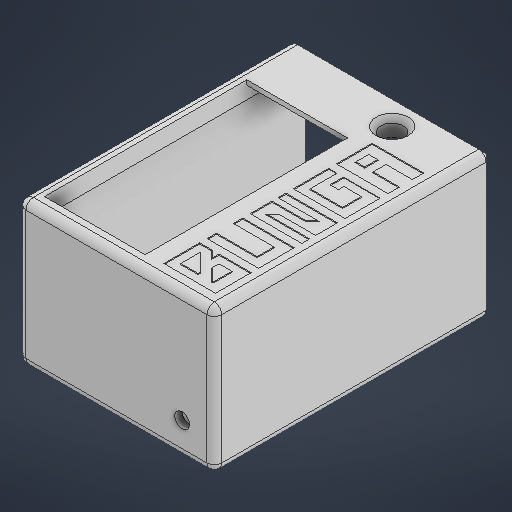
# Autodesk Inventor part: PowerSupplyRegulator-OnePiece
Saved by Autodesk Inventor 2026.2 (Build 302298010, 298A)
## iProperties
Created: 2026-07-26
Part Number: PowerSupplyRegulator-OnePiece
Material: Generic
Document SubType Name: Modeling
Designer: incep
Density: 1 g/cm^3
Appearance: Default
Author: incep
## iProperties of the stored document PowerSupplyRegulator-OnePiece_3DPrint.ipt
Created: 2026-07-26
Part Number: PowerSupplyRegulator-OnePiece_3DPrint
Material: Generic
Document SubType Name: Modeling
Designer: incep
Density: 1 g/cm^3
Appearance: Default
Author: incep
Autodesk Inventor part; units mm, degrees
ref_plane "YZ Plane" through (0, 0, 0) normal (1, 0, 0) x (0, 1, 0)
ref_plane "XZ Plane" through (0, 0, 0) normal (0, 1, 0) x (-1, 0, 0)
ref_plane "XY Plane" through (0, 0, 0) normal (0, 0, 1) x (1, 0, 0)
sketch "Sketch1" plane through (0, 0, 0) normal (0, 0, 1) x (1, 0, 0)
  line L0 (-36.5, 21.9) -> (36.5, 21.9)
  line L1 (36.5, 21.9) -> (36.5, -21.9)
  line L2 (36.5, -21.9) -> (-36.5, -21.9)
  line L3 (-36.5, -21.9) -> (-36.5, 21.9)
  line L4 (-39.5, 28.9) -> (39.5, 28.9)
  line L5 (39.5, 28.9) -> (39.5, -28.9)
  line L6 (39.5, -28.9) -> (-39.5, -28.9)
  line L7 (-39.5, -28.9) -> (-39.5, 28.9)
  point P0 (0, 0)
  point P1 (36.5, 0)
  point P2 (0, 21.9)
  point P3 (0, 28.9)
  point P4 (39.5, 0)
  dimension "d0" = 73
  dimension "d1" = 43.8
  dimension "d2" = 3
  dimension "d3" = 7
  constraints: 16 end point, 4 midpoint, 4 parallel, 2 horizontal, 2 horizontal alignment, 2 perpendicular, 2 vertical alignment
  measures "d0" distance of L0.start L0.end
  measures "d1" distance of L2.end L0.start
  measures "d2" distance between parallel lines of L7 L3
  measures "d3" distance between parallel lines of L4 L0
extrude "Extrusion1" add sketch "Sketch1" along normal blind 109.6
sketch "Sketch3" plane through (0, 0, 109.6) normal (0, 0, 1) x (1, 0, 0)
  point P0 (0, 0)
sketch "Sketch2" plane through (0, 0, 109.6) normal (0, 0, 1) x (1, 0, 0)
  line L0 (39.5, -28.9) -> (39.5, 28.9) projected
  line L1 (39.5, 28.9) -> (-39.5, 28.9) projected
  line L2 (-39.5, 28.9) -> (-39.5, -28.9) projected
  line L3 (-39.5, -28.9) -> (39.5, -28.9) projected
  point P0 (0, 0)
sketch "Sketch4" plane through (0, 0, 109.6) normal (0, 0, 1) x (1, 0, 0)
  line L0 (-36.5, 27) -> (36.5, 27)
  line L1 (36.5, 27) -> (36.5, -27)
  line L2 (36.5, -27) -> (-36.5, -27)
  line L3 (-36.5, -27) -> (-36.5, 27)
  line L4 (-36.5, -21.9) -> (-36.5, 21.9) projected
  line L5 (39.5, 28.9) -> (-39.5, 28.9) projected
  point P0 (0, 0)
  point P1 (36.5, 0)
  point P2 (0, 27)
  dimension "d6" = 54
  dimension "d43" = 1.9
  constraints: 8 end point, 2 midpoint, 2 parallel, 1 collinear, 1 horizontal, 1 horizontal alignment, 1 perpendicular, 1 vertical alignment
  measures "d6" distance between parallel lines of L2 L0
  measures "d43" distance between parallel lines of L5 L0
extrude "Extrusion2" cut sketch "Sketch4" against normal blind 86.6
sketch "Sketch6" plane through (-39.5, 28.9, 0) normal (0, 1, 0) x (1, 0, 0)
  line L0 (3, -109.6) -> (76, -109.6) projected
  line L1 (3, -109.6) -> (3, -23) projected
  line L2 (3, -23) -> (76, -23) projected
  line L3 (76, -109.6) -> (76, -23) projected
  line L4 (45.6, -25.5) -> (5, -25.5)
  line L5 (5, -25.5) -> (5, -107.1)
  line L6 (5, -107.1) -> (45.6, -107.1)
  line L7 (45.6, -107.1) -> (45.6, -25.5)
  point P0 (39.5, 0)
  point P1 (45.6, -66.3)
  point P2 (76, -66.3)
  point P3 (25.3, -25.5)
  point P4 (39.5, -23)
  dimension "d9" = 81.6
  dimension "d10" = 40.6
  dimension "d11" = 2
  dimension "d20" = 2.5
  constraints: 8 end point, 4 midpoint, 2 parallel, 1 horizontal, 1 perpendicular
  measures "d9" distance of L6.end L4.start
  measures "d10" distance between parallel lines of L5 L7
  measures "d11" distance between parallel lines of L1 L5
  measures "d20" distance between parallel lines of L0 L6
extrude "Extrusion3" cut sketch "Sketch6" against normal up to surface (1.9 mm away) contours L7 L6 L5 L4
sketch "Sketch7" plane through (-36.5, -21.9, 0) normal (0, 1, 0) x (1, 0, 0)
  circle A0 centre (62.3, -14.3) radius 5.25
  circle A1 centre (10.7, -14.3) radius 5.25
  line L0 (62.3, -14.3) -> (10.7, -14.3) construction
  line L1 (73, 0) -> (0, 0) construction
  point P0 (36.5, 0)
  point P1 (36.5, 0)
  point P2 (36.5, -14.3)
  dimension "d14" = 51.6
  dimension "d15" = 10.5
  dimension "d16" = 14.3
  constraints: 2 centre point, 2 end point, 2 midpoint, 1 equal radius, 1 horizontal, 1 vertical alignment
  measures "d14" distance of L0.start L0.end
  measures "d15" diameter of A0
  measures "d16" distance between parallel lines of L0 L1
extrude "Extrusion4" cut sketch "Sketch7" against normal blind 0.9
fillet "Fillet1" [suppressed]
chamfer "Chamfer1" distance 3 angle 45 2 edges at (0, 21.9, 23) (0, -21.9, 23)
chamfer "Chamfer2" distance 2 angle 45 1 edges at (0, -21.9, 0)
sketch "Sketch8" plane through (-39.5, -25.95, 0) normal (-1, 0, 0) x (0, 0, 1)
  line L0 (2, 4.05) -> (20, 4.05) projected
  line L1 (2, 4.05) -> (20, 4.05) projected
  line L2 (9.05, 4.05) -> (19.55, 4.05) projected
  line L3 (9.05, 4.05) -> (19.55, 4.05) projected
  circle A0 centre (8.5, 1) radius 2.1
  line L4 (0, -2.95) -> (109.6, -2.95) projected
  line L5 (0, -2.95) -> (109.6, -2.95) projected
  point P0 (0, 25.95)
  point P1 (8.5, 4)
  point P2 (8.5, 4)
  dimension "d27" = 4.2
  dimension "d28" = 3
  constraints: 1 centre point, 1 vertical alignment, 4 other
  measures "d27" diameter of A0
  measures "d28" distance of A0.centre point (8.5, 4)
extrude "Extrusion5" [suppressed]
sketch "Sketch9" plane through (-33.5, -24.95, 8.5) normal (-1, 0, 0) x (0, 0, 1)
  circle A0 centre (0, 0) radius 2.1 projected
  circle A1 centre (0, 0) radius 1.7
  point P0 (-8.5, 24.95)
  dimension "d31" = 3.4
  constraints: 1 centre point, 1 coincident
  measures "d31" diameter of A1
extrude "Extrusion6" [suppressed]
sketch "Sketch10" plane through (39.5, -25.95, 0) normal (1, 0, 0) x (0, 0, -1)
  point P0 (0, 25.95)
sketch "Sketch11" plane through (39.5, -25.95, 0) normal (1, 0, 0) x (0, 0, -1)
  circle A0 centre (-8.5, 1) radius 1.7 projected
  circle A1 centre (-8.5, 1) radius 3
  point P0 (0, 25.95)
  dimension "d34" = 6
  constraints: 1 centre point, 1 coincident
  measures "d34" diameter of A1
extrude "Extrusion7" add sketch "Sketch2" along normal blind 3
fillet "Fillet2" [suppressed]
sketch "Sketch12" plane through (0, 0, 112.6) normal (0, 0, 1) x (1, 0, 0)
  circle A0 centre (26.5, -15.95) radius 3
  line L0 (36.5, 25.95) -> (36.5, -25.95) projected
  line L1 (36.5, -25.95) -> (-36.5, -25.95) projected
  point P0 (0, 0)
  dimension "d38" = 6
  dimension "d39" = 10
  dimension "d40" = 10
  constraints: 1 centre point
  measures "d38" diameter of A0
  measures "d39" distance from line of L0 A0.centre
  measures "d40" distance from line of L1 A0.centre
extrude "Extrusion8" cut sketch "Sketch12" against normal up to surface (3 mm away)
fillet "Fillet3" radius 3 8 edges at (-39.5, -28.9, 56.3) (-39.5, 28.9, 56.3) (39.5, -28.9, 56.3) (39.5, 28.9, 56.3) (0, 28.9, 112.6) (39.5, 0, 112.6) (0, -28.9, 112.6) (-39.5, 0, 112.6)
fillet "Fillet4" radius 6 4 edges at (36.5, -21.9, 11) (36.5, 21.9, 10) (-36.5, -21.9, 11) (-36.5, 21.9, 10)
sketch "Sketch13" plane through (-36.5, 28.9, 0) normal (0, 1, 0) x (1, 0, 0)
  line L0 (0, -23) -> (73, -23) projected
  line L1 (0, -14) -> (0, 0) projected
  line L2 (0, -23) -> (0, -14) projected
  line L3 (0, -109.6) -> (0, -23) projected
  line L4 (0, -109.6) -> (0, -23) projected
  line L5 (0, -14) -> (0, -23) projected
  line L6 (0, -8) -> (0, -14) projected
  line L7 (0, 0) -> (0, -8) projected
  line L8 (73, 0) -> (73, -14) projected
  line L9 (73, -8) -> (73, 0) projected
  line L10 (73, -14) -> (73, -8) projected
  line L11 (73, -23) -> (73, -14) projected
  line L12 (73, -109.6) -> (73, -23) projected
  line L13 (73, -109.6) -> (73, -23) projected
  line L14 (73, -14) -> (73, -23) projected
  circle A0 centre (47.6, -12.5) radius 4.5
  point P0 (36.5, 0)
  dimension "d46" = 9
  dimension "d47" = 25.4
  dimension "d48" = 10.5
  constraints: 1 centre point
  measures "d46" diameter of A0
  measures "d47" distance from line of A0.centre L11
  measures "d48" distance from line of L0 A0.centre
extrude "Extrusion9" cut sketch "Sketch13" against normal up to surface (7 mm away)
chamfer "Chamfer3" distance 2 angle 45 1 edges at (6.6, 28.9, 12.5)
chamfer "Chamfer4" distance 3 angle 45 8 edges at (0, 28.9, 0) (-38.6213, 28.0213, 0) (-39.5, 0, 0) (-38.6213, -28.0213, 0) (0, -28.9, 0) (38.6213, -28.0213, 0) (39.5, 0, 0) (38.6213, 28.0213, 0)
sketch "Sketch14" plane through (-36.5, 28.9, 109.6) normal (0, 1, 0) x (1, 0, 0)
  line L0 (70.0467, 55.6168) -> (49.6467, 55.6168) construction
  line L1 (49.6467, 52.2168) -> (70.0467, 52.2168) construction
  line L2 (49.6467, 55.6168) -> (49.6467, 69.6168) construction
  line L3 (49.6467, 55.6168) -> (70.0467, 55.6168)
  line L4 (49.6467, 69.6168) -> (49.6467, 55.6168)
  line L5 (70.0467, 69.6168) -> (70.0467, 55.6168) construction
  line L6 (49.6467, 69.6168) -> (70.0467, 69.6168) construction
  line L7 (70.0467, 55.6168) -> (49.6467, 55.6168) construction
  line L8 (55.6467, 64.4168) -> (58.6467, 64.4168)
  line L9 (58.6467, 64.4168) -> (58.6467, 66.6168)
  line L10 (66.0467, 66.6168) -> (66.0467, 58.6168)
  line L11 (58.6467, 66.6168) -> (66.0467, 66.6168)
  line L12 (52.6467, 58.6168) -> (52.6467, 69.6168)
  line L13 (55.6467, 69.6168) -> (55.6467, 64.4168)
  line L14 (70.0467, 55.6168) -> (70.0467, 69.6168)
  line L15 (70.0467, 69.6168) -> (55.6467, 69.6168)
  line L16 (66.0467, 58.6168) -> (52.6467, 58.6168)
  line L17 (49.6467, 69.6168) -> (70.0467, 69.6168) construction
  line L18 (70.0467, 73.0168) -> (49.6467, 73.0168) construction
  line L19 (49.6467, 87.0168) -> (70.0467, 87.0168) construction
  line L20 (49.6467, 73.0168) -> (49.6467, 87.0168) construction
  line L21 (70.0467, 87.0168) -> (70.0467, 73.0168) construction
  line L22 (52.6467, 69.6168) -> (49.6467, 69.6168)
  line L23 (49.6467, 73.0168) -> (70.0467, 73.0168)
  line L24 (70.0467, 73.0168) -> (70.0467, 77.2168)
  line L25 (70.0467, 77.2168) -> (59.4467, 77.2168)
  line L26 (52.4467, 77.2168) -> (56.4467, 77.2168)
  line L27 (59.4467, 77.2168) -> (59.4467, 82.8168)
  line L28 (59.4467, 82.8168) -> (70.0467, 82.8168)
  line L29 (70.0467, 82.8168) -> (70.0467, 87.0168)
  line L30 (70.0467, 87.0168) -> (49.6467, 87.0168)
  line L31 (49.6467, 87.0168) -> (49.6467, 73.0168)
  line L32 (56.4467, 82.8168) -> (52.4467, 82.8168)
  line L33 (52.4467, 82.8168) -> (52.4467, 77.2168)
  line L34 (56.4467, 77.2168) -> (56.4467, 82.8168)
  line L35 (70.0467, 38.2168) -> (49.6467, 38.2168) construction
  line L36 (49.6467, 34.8168) -> (70.0467, 34.8168) construction
  line L37 (49.6467, 34.8168) -> (70.0467, 34.8168) construction
  line L38 (70.0467, 34.8168) -> (70.0467, 20.8168) construction
  line L39 (70.0467, 20.8168) -> (49.6467, 20.8168) construction
  line L40 (49.6467, 20.8168) -> (49.6467, 34.8168) construction
  line L41 (49.6467, 20.8168) -> (49.6467, 34.8168) construction
  line L42 (70.0467, 52.2168) -> (70.0467, 38.2168) construction
  line L43 (49.6467, 38.2168) -> (49.6467, 52.2168) construction
  line L44 (49.6467, 52.2168) -> (70.0467, 52.2168) construction
  line L45 (70.0467, 38.2168) -> (49.6467, 38.2168) construction
  line L46 (70.0467, 52.2168) -> (70.0467, 38.2168) construction
  line L47 (49.6467, 38.2168) -> (49.6467, 52.2168) construction
  line L48 (49.6467, 55.6168) -> (49.6467, 69.6168) construction
  line L49 (70.0467, 69.6168) -> (70.0467, 55.6168) construction
  line L50 (49.6467, 38.2168) -> (49.6467, 52.2168) construction
  line L51 (70.0467, 41.0168) -> (70.0467, 38.2168)
  line L52 (55.4467, 43.8168) -> (52.6467, 41.0168)
  line L53 (49.6467, 46.6168) -> (63.2467, 46.6168)
  line L54 (66.0467, 49.4168) -> (49.6467, 49.4168)
  line L55 (49.6467, 52.2168) -> (70.0467, 52.2168) construction
  line L56 (49.6467, 52.2168) -> (70.0467, 52.2168)
  line L57 (70.0467, 38.2168) -> (49.6467, 38.2168)
  line L58 (70.0467, 38.2168) -> (49.6467, 38.2168) construction
  line L59 (52.6467, 41.0168) -> (70.0467, 41.0168)
  line L60 (70.0467, 43.8168) -> (55.4467, 43.8168)
  line L61 (63.2467, 46.6168) -> (66.0467, 49.4168)
  line L62 (70.0467, 52.2168) -> (70.0467, 38.2168) construction
  line L63 (70.0467, 52.2168) -> (70.0467, 43.8168)
  line L64 (70.0467, 34.8168) -> (70.0467, 20.8168) construction
  line L65 (59.8467, 15.3688) -> (59.8467, 15.3688)
  line L66 (49.6467, 17.4168) -> (54.4376, 17.4168)
  line L67 (53.171, 14.4168) -> (52.6467, 14.4168)
  line L68 (54.4376, 17.4168) -> (57.4376, 14.4168)
  line L69 (57.4376, 14.4168) -> (57.4376, 17.4168)
  line L70 (59.8467, 15.3688) -> (59.8467, 17.4168) construction
  line L71 (59.8467, 15.3688) -> (59.8467, 17.4168) construction
  line L72 (57.4376, 14.4168) -> (60.4376, 11.4168) construction
  line L73 (60.4376, 11.4168) -> (60.4376, 14.4168)
  line L74 (60.4376, 14.4168) -> (66.0467, 14.4168)
  line L75 (70.0467, 17.4168) -> (57.4376, 17.4168)
  line L76 (49.6467, 34.8168) -> (70.0467, 34.8168)
  line L77 (66.0467, 31.4168) -> (49.6467, 31.4168)
  line L78 (66.0467, 24.2168) -> (66.0467, 31.4168)
  line L79 (70.0467, 34.8168) -> (70.0467, 20.8168)
  line L80 (49.6467, 24.2168) -> (66.0467, 24.2168)
  line L81 (49.6467, 20.8168) -> (49.6467, 24.2168)
  line L82 (70.0467, 20.8168) -> (49.6467, 20.8168)
  line L83 (49.6467, 17.4168) -> (49.6467, 3.4168)
  line L84 (70.0467, 3.4168) -> (70.0467, 17.4168)
  line L85 (49.6467, 17.4168) -> (70.0467, 17.4168) construction
  line L86 (49.6467, 3.4168) -> (49.6467, 17.4168) construction
  line L87 (70.0467, 3.4168) -> (49.6467, 3.4168) construction
  line L88 (70.0467, 17.4168) -> (70.0467, 3.4168) construction
  line L89 (70.0467, 20.8168) -> (49.6467, 20.8168) construction
  line L90 (52.6467, 6.4168) -> (60.0715, 6.4168)
  line L91 (56.3591, 6.4168) -> (56.3591, 11.945) construction
  line L92 (60.0715, 6.4168) -> (60.0715, 7.5163)
  line L93 (66.0467, 14.4168) -> (66.0467, 6.4168)
  line L94 (66.0467, 6.4168) -> (65.4376, 6.4168)
  line L95 (65.4376, 6.4168) -> (60.4376, 11.4168)
  line L96 (60.0715, 7.5163) -> (53.171, 14.4168)
  line L97 (52.6467, 14.4168) -> (52.6467, 6.4168)
  line L98 (65.4376, 6.4168) -> (65.4376, 0.7147) construction
  line L99 (49.6467, 3.4168) -> (70.0467, 3.4168)
  line L100 (49.6467, 52.2168) -> (49.6467, 49.4168)
  line L101 (49.6467, 46.6168) -> (49.6467, 38.2168)
  line L102 (49.6467, 34.8168) -> (49.6467, 31.4168)
  point P0 (36.5, 109.6)
  point P1 (48.2467, 45.2168)
  point P2 (49.6467, 62.6168)
  point P3 (49.6467, 62.6168)
  point P4 (59.8467, 52.2168)
  point P5 (59.8467, 62.6168)
  point P6 (59.8467, 69.6168)
  point P7 (59.8467, 69.6168)
  point P8 (49.6467, 80.0168)
  point P9 (59.8467, 80.0168)
  point P10 (59.8467, 87.0168)
  point P11 (49.6467, 45.2168)
  point P12 (59.8467, 45.2168)
  point P13 (59.8467, 34.8168)
  point P14 (59.8467, 34.8168)
  point P15 (49.6467, 27.8168)
  point P16 (49.6467, 27.8168)
  point P17 (49.6467, 45.2168)
  point P18 (59.8467, 62.6168)
  point P19 (59.8467, 53.2168)
  point P20 (59.8467, 52.2168)
  point P21 (59.8467, 45.2168)
  point P22 (49.6467, 45.2168)
  point P23 (59.8467, 45.2168)
  point P24 (59.8467, 52.2168)
  point P25 (59.8467, 45.2168)
  point P26 (55.6986, 19.5168)
  point P27 (59.8467, 17.4168)
  point P28 (49.6467, 10.4168)
  point P29 (59.8467, 10.4168)
  point P30 (59.8467, 27.8168)
  point P31 (59.8467, 27.8168)
  point P32 (61.4467, 45.2168)
  point P33 (61.4467, 45.2168)
  constraints: 206 end point, 27 perpendicular, 17 collinear, 17 point on line, 6 midpoint, 4 parallel, 2 coincident
extrude "Extrusion10" cut sketch "Sketch14" against normal blind 0.2
chamfer "Chamfer5" distance 0.2 angle 45 58 edges at (13.1467, 28.9, 99.1832) (15.5421, 28.9, 92.1832) (23.3467, 28.9, 106.1832) (33.5467, 28.9, 99.1832) (27.2421, 28.9, 92.1832) (20.9376, 28.9, 93.6832) (19.4376, 28.9, 93.6832) (20.1212, 28.9, 98.6334) (23.5715, 28.9, 102.6334) (19.8591, 28.9, 103.1832) (16.1467, 28.9, 99.1832) (26.4376, 28.9, 100.6832) (23.9376, 28.9, 96.6832) (26.7421, 28.9, 95.1832) (29.5467, 28.9, 99.1832) (29.2421, 28.9, 103.1832) (23.3467, 28.9, 88.7832) (13.1467, 28.9, 87.0832) (21.3467, 28.9, 85.3832) (21.3467, 28.9, 78.1832) (13.1467, 28.9, 76.4832) (23.3467, 28.9, 74.7832) (33.5467, 28.9, 81.7832) (29.5467, 28.9, 81.7832) (13.1467, 28.9, 67.1832) (23.3467, 28.9, 71.3832) (24.8467, 28.9, 68.5832) (17.5467, 28.9, 67.1832) (26.2467, 28.9, 65.7832) (33.5467, 28.9, 69.9832) (33.5467, 28.9, 61.5832) (19.9467, 28.9, 62.9832) (28.1467, 28.9, 61.5832) (21.3467, 28.9, 60.1832) (13.1467, 28.9, 58.7832) (23.3467, 28.9, 57.3832) (13.1467, 28.9, 46.9832) (23.3467, 28.9, 53.9832) (22.8467, 28.9, 50.9832) (16.1467, 28.9, 45.4832) (19.1467, 28.9, 42.5832) (20.6467, 28.9, 45.1832) (22.1467, 28.9, 44.0832) (25.8467, 28.9, 42.9832) (29.5467, 28.9, 46.9832) (33.5467, 28.9, 46.9832) (23.3467, 28.9, 36.5832) (13.1467, 28.9, 29.5832) (23.3467, 28.9, 22.5832) (19.9467, 28.9, 29.5832) (17.9467, 28.9, 32.3832) (15.9467, 28.9, 29.5832) (17.9467, 28.9, 26.7832) (22.9467, 28.9, 29.5832) (28.2467, 28.9, 32.3832) (28.2467, 28.9, 26.7832) (33.5467, 28.9, 24.6832) (33.5467, 28.9, 34.4832)
sketch "Sketch15" plane through (-36.5, 27, 23) normal (0, -1, 0) x (1, 0, 0)
  line L0 (42.6, -3) -> (73, -3)
  line L1 (73, -3) -> (73, 86.6)
  line L2 (73, 86.6) -> (42.6, 86.6)
  line L3 (42.6, 86.6) -> (42.6, -3)
  line L4 (42.6, 84.1) -> (42.6, 2.5) projected
  line L5 (0, 86.6) -> (73, 86.6) projected
  line L6 (6, -3) -> (67, -3) projected
  line L7 (73, 86.6) -> (73, 0) projected
  line L8 (0, 86.6) -> (2, 86.6)
  line L9 (2, 86.6) -> (2, -3)
  line L10 (2, -3) -> (0, -3)
  line L11 (0, -3) -> (0, 86.6)
  line L12 (0, 86.6) -> (0, 0) projected
  line L13 (2, 2.5) -> (2, 84.1) projected
  point P0 (36.5, -23)
  point P1 (2, 86.6)
  constraints: 16 end point, 8 collinear, 4 parallel, 2 horizontal, 2 perpendicular
extrude "Extrusion11" add sketch "Sketch15" along normal up to surface (5.1 mm away)
sketch "Sketch16" plane through (-36.5, -27, 23) normal (0, 1, 0) x (1, 0, 0)
  line L0 (73, -86.6) -> (0, -86.6)
  line L1 (0, -86.6) -> (0, 3)
  line L2 (0, 3) -> (73, 3)
  line L3 (73, 3) -> (73, -86.6)
  line L4 (73, -86.6) -> (0, -86.6) projected
  line L5 (0, -86.6) -> (0, 0) projected
  line L6 (73, -86.6) -> (73, 0) projected
  line L7 (67, 3) -> (6, 3) projected
  point P0 (36.5, 23)
  constraints: 8 end point, 4 collinear, 2 parallel, 1 horizontal, 1 perpendicular
extrude "Extrusion12" add sketch "Sketch16" along normal blind 0.7
body "Solid1"
